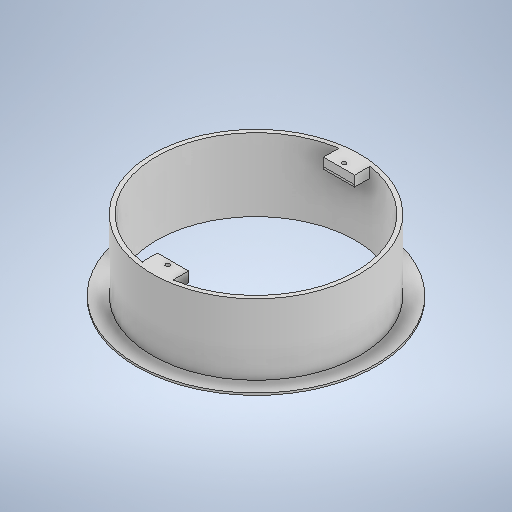
# Autodesk Inventor part: Chassis_Support
Saved by Autodesk Inventor 2025 (Build 290162000, 162)
## iProperties
Created: 2024-06-28
Part Number: Chassis_Support
Material: Generic
Document SubType Name: Modeling
Designer: sml6042
Density: 1 g/cm^3
Appearance: Default
Author: sml6042
Autodesk Inventor part; units mm, degrees
ref_plane "YZ Plane" through (0, 0, 0) normal (1, 0, 0) x (0, 1, 0)
ref_plane "XZ Plane" through (0, 0, 0) normal (0, 1, 0) x (-1, 0, 0)
ref_plane "XY Plane" through (0, 0, 0) normal (0, 0, 1) x (1, 0, 0)
sketch "Sketch1" plane through (0, 0, 0) normal (0, 1, 0) x (-1, 0, 0)
  circle A0 centre (0, 0) radius 57.5
  circle A1 centre (0, 0) radius 48
  circle A2 centre (0, 0) radius 50
  line L0 (0, 0) -> (7.5, 0)
  line L1 (7.5, 0) -> (-7.5, 0)
  line L2 (-7.5, 0) -> (-7.5, -47.4104)
  line L3 (7.5, 0) -> (7.5, -47.4104)
  line L4 (7.5, 0) -> (7.5, 47.4104)
  line L5 (-7.5, 0) -> (-7.5, 47.4104)
  dimension "d0" = 115
  dimension "d1" = 96
  dimension "d2" = 100
  constraints: 12 end point, 4 point on circle, 3 centre point, 3 coincident, 3 equal length, 1 horizontal, 1 point on line, 1 vertical
  measures "d0" diameter of A0
  measures "d1" diameter of A1
  measures "d2" diameter of A2
extrude "Extrusion1" add sketch "Sketch1" along normal blind 1 contours A0 | A1 L3 L4 | L4 L0 L1 L5 A1 | A1 L2 L1 L0 L3 | L5 L2 A1 | A2
sketch "Sketch2" plane through (0, 1, 0) normal (0, 1, 0) x (1, 0, 0)
  circle A0 centre (0, 0) radius 49
  circle A1 centre (0, 0) radius 50
  line L0 (0, 0) -> (7.5, 0)
  line L1 (7.5, -48.4226) -> (7.5, 48.4226) projected
  line L2 (7.5, 0) -> (7.5, 48.4226)
  line L3 (7.5, 48.4226) -> (7.5, -48.4226)
  line L4 (-7.5, 48.4226) -> (-7.5, -48.4226)
  dimension "d7" = 98
  dimension "d8" = 100
  constraints: 8 end point, 3 point on circle, 2 centre point, 2 coincident, 1 collinear, 1 midpoint, 1 parallel, 1 point on line
  measures "d7" diameter of A0
  measures "d8" diameter of A1
extrude "Extrusion2" add sketch "Sketch2" along normal blind 30 contours L1 A0 L4 | A1
sketch "Sketch3" plane through (0, 0, 0) normal (0, -1, 0) x (1, 0, 0)
  circle A0 centre (0, 0) radius 49
  line L0 (0, 0) -> (0, 40)
  line L1 (0, 40) -> (0, -40)
  dimension "d11" = 98
  dimension "d12" = 40
  dimension "d13" = 80
  constraints: 4 end point, 1 centre point, 1 coincident, 1 point on line, 1 vertical
  measures "d11" diameter of A0
  measures "d12" distance of L0.start L0.end
  measures "d13" distance of L0.end L1.end
extrude "Extrusion3" cut sketch "Sketch3" against normal blind 30
sketch "Sketch4" plane through (0, 31, 0) normal (0, 1, 0) x (1, 0, 0)
  line L0 (0, 0) -> (0, -40)
  line L1 (0, -40) -> (-7.5, -40)
  line L2 (-7.5, 48.4226) -> (-7.5, -48.4226) projected
  line L3 (7.5742, -40) -> (0, -40)
  line L4 (7.5742, -40) -> (7.5, 40)
  line L5 (7.5, -48.4226) -> (7.5, 48.4226) projected
  line L6 (7.5, 40) -> (-7.5742, 39.986)
  line L7 (-7.5742, 39.986) -> (-7.5, -40)
  line L8 (-7.5, -40) -> (-7.5742, 39.986)
  line L9 (0, -40) -> (0, -42.5)
  line L10 (-0.0371, 39.993) -> (-0.0371, 42.493)
  circle A0 centre (-0.0371, 42.493) radius 1.025
  circle A1 centre (0, -42.5) radius 1.025
  point P0 (-7.5, 39.9861)
  point P1 (7.5, -40)
  dimension "d16" = 40
  dimension "d17" = 80
  dimension "d18" = 2.5
  dimension "d19" = 2.5
  dimension "d20" = 2.05
  dimension "d21" = 2.05
  constraints: 18 end point, 4 point on line, 3 perpendicular, 2 centre point, 2 coincident, 2 collinear, 2 vertical, 1 midpoint
  measures "d16" distance of L0.start L0.end
  measures "d17" distance of L3.start L4.end
  measures "d18" distance of L0.end L9.end
  measures "d19" distance of L10.start L10.end
  measures "d20" diameter of A0
  measures "d21" diameter of A1
extrude "Extrusion4" cut sketch "Sketch4" against normal through all contours L1 L2 L6 L5 L3 | A0 | A1
sketch "Sketch5" plane through (0, 0, 0) normal (0, -1, 0) x (1, 0, 0)
  circle A0 centre (0, 0) radius 49
  circle A1 centre (0, 0) radius 48
  dimension "d24" = 98
  dimension "d25" = 96
  constraints: 2 centre point, 2 coincident
  measures "d24" diameter of A0
  measures "d25" diameter of A1
extrude "Extrusion5" add sketch "Sketch5" against normal blind 31
sketch "Sketch6" plane through (0, 31, 0) normal (0, 1, 0) x (1, 0, 0)
  circle A0 centre (0, 0) radius 50
  circle A1 centre (0, -42.5) radius 1.025 projected
  circle A2 centre (0, -42.5) radius 1.025
  line L0 (-7.5, -40) -> (-7.5, -47.4104) projected
  line L1 (-7.5, -47.4104) -> (-7.5, -40)
  line L2 (7.5, -47.4104) -> (7.5, -40) projected
  line L3 (-7.5, -40) -> (7.5, -40)
  line L4 (7.5, -40) -> (-7.5, -40)
  line L5 (-7.5, -47.4104) -> (-7.5, -40)
  line L6 (7.5, -40) -> (-7.5, -40)
  arc A3 (7.5, -47.4104) -> (7.5, 47.4104) centre (0, 0) ccw
  arc A4 (-7.5, 47.4104) -> (-7.5, -47.4104) centre (0, 0) ccw
  line L7 (7.5, 40) -> (7.5, 47.4104) projected
  line L8 (7.5, 47.4104) -> (7.5, 40)
  line L9 (7.5, 40) -> (-7.5, 40)
  line L10 (-7.5, 40) -> (-7.5, 47.4104)
  circle A5 centre (-0.0371, 42.493) radius 1.025 projected
  circle A6 centre (-0.0371, 42.493) radius 1.025
  dimension "d28" = 100
  dimension "d30" = 2.05
  dimension "d31" = 2.05
  constraints: 17 end point, 6 perpendicular, 5 centre point, 4 coincident, 4 point on circle, 2 collinear, 2 point on line
  measures "d28" diameter of A0
  measures "d30" diameter of A2
  measures "d31" diameter of A6
extrude "Extrusion6" add sketch "Sketch6" along normal blind 4
body "Solid1"
